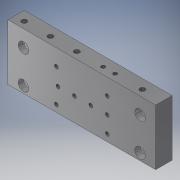
# Autodesk Inventor part: XcolBracket
Saved by Autodesk Inventor 2019 (Build 230136000, 136)
## iProperties
Created: 2018-10-03
Part Number: XcolBracket
Material: Aluminum 6061-AHC
Document SubType Name: Modeling
Designer: LillaHunden
Mass: 97.2 g
Surface Area: 98 cm^2
Volume: 36 cm^3
Density: 2.7 g/cm^3
Appearance: Aluminum - Dark
Author: LillaHunden
Autodesk Inventor part; units mm, degrees
ref_plane "YZ Plane" through (0, 0, 0) normal (1, 0, 0) x (0, 1, 0)
ref_plane "XZ Plane" through (0, 0, 0) normal (0, 1, 0) x (-1, 0, 0)
ref_plane "XY Plane" through (0, 0, 0) normal (0, 0, 1) x (1, 0, 0)
sketch "Sketch1" plane through (0, 0, 0) normal (0, 0, 1) x (1, 0, 0)
  line L0 (22.4756, 14.1051) -> (-67.5244, 14.1051)
  line L1 (-67.5244, 14.1051) -> (-67.5244, -22.9199)
  line L2 (-67.5244, -22.9199) -> (22.4756, -22.9199)
  line L3 (22.4756, -22.9199) -> (22.4756, 14.1051)
  point P0 (0, 0)
  dimension "d0" = 90
  constraints: 8 end point, 2 parallel, 1 horizontal, 1 perpendicular
  measures "d0" distance of L2.end L1.end
extrude "Extrusion1" add sketch "Sketch1" along normal blind 10
sketch "Sketch2" plane through (0, 0, 10) normal (0, 0, 1) x (1, 0, 0)
  point P0 (12.9756, 4.1051)
  point P1 (12.9756, -15.8949)
  point P2 (-58.0244, 4.1051)
  point P3 (-58.0244, -15.8949)
hole "Hole1" at (12.9756, 4.1051, 10) at (12.9756, -15.8949, 10) at (-58.0244, 4.1051, 10) at (-58.0244, -15.8949, 10) direction (0, 0, -1) diameter 3.4 depth 10 counterbore diameter 6.5 counterbore depth 3.4
sketch "Sketch3" plane through (-67.5244, 14.1051, 0) normal (0, 1, 0) x (1, 0, 0)
  point P0 (61.1484, -15)
  point P1 (53.8516, -15)
  point P2 (61.15, -5.8303)
  point P3 (53.85, -5.8303)
hole "Hole3" at (-6.376, 14.1051, 15) at (-13.6728, 14.1051, 15) at (-6.3744, 14.1051, 5.8303) at (-13.6744, 14.1051, 5.8303) direction (0, -1, 0) diameter 2.459 depth 10.4 tip angle 120 thread size "M3x0.5" class "6H" standard "ISO Metric profile"
sketch "Sketch4" plane through (-67.5244, 14.1051, 0) normal (0, 1, 0) x (1, 0, 0)
  point P0 (37.7681, -15)
  point P1 (37.7681, -5.8303)
  point P2 (21.7681, -5.8303)
  point P3 (5.7681, -5.8303)
  point P4 (77.7681, -5.8303)
hole "Hole5" at (-29.7563, 14.1051, 15) at (-29.7563, 14.1051, 5.8303) at (-45.7563, 14.1051, 5.8303) at (-61.7563, 14.1051, 5.8303) at (10.2437, 14.1051, 5.8303) direction (0, -1, 0) diameter 3.242 depth 10.5 tip angle 120 thread size "M4x0.7" class "6H" standard "ISO Metric profile"
sketch "Sketch7" plane through (0, 0, 10) normal (0, 0, 1) x (1, 0, 0)
  point P0 (-7.0244, -15.8949)
  point P1 (-7.0244, 4.1051)
  point P2 (-38.0244, -15.8949)
  point P3 (-38.0244, 4.1051)
hole "Hole10" at (-7.0244, -15.8949, 10) at (-7.0244, 4.1051, 10) at (-38.0244, -15.8949, 10) at (-38.0244, 4.1051, 10) direction (0, 0, -1) diameter 2.459 depth 8.4 tip angle 120 thread size "M3x0.5" class "6H" standard "ISO Metric profile"
sketch "Sketch8" plane through (0, 0, 10) normal (0, 0, 1) x (1, 0, 0)
  point P0 (-7.0244, -5.8949)
  point P1 (-17.0244, -5.8949)
  point P2 (-27.0244, -5.8949)
  point P3 (-37.0244, -5.8949)
hole "Hole12" at (-7.0244, -5.8949, 10) at (-17.0244, -5.8949, 10) at (-27.0244, -5.8949, 10) at (-37.0244, -5.8949, 10) direction (0, 0, -1) diameter 2.459 depth 8.4 tip angle 120 thread size "M3x0.5" class "6H" standard "ISO Metric profile"
body "Solid1"
